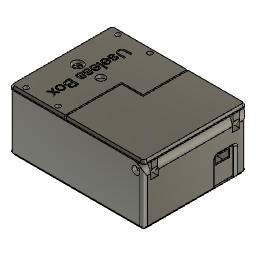
Smart_Useless_Box_box_v2 (Autodesk Fusion 360 design; units mm, degrees)
Autodesk Fusion 360 part; units mm, degrees
(part 1 of 2)
sketch "Base" plane through (0, 0, 0) normal (0, 0, 1) x (1, 0, 0) in component "Box Base"
  line L0 (50, -37.5) -> (-50, -37.5)
  line L1 (-50, -37.5) -> (-50, 37.5)
  line L2 (-50, 37.5) -> (50, 37.5)
  line L3 (50, 37.5) -> (50, -37.5)
  line L4 (50, -37.5) -> (-50, 37.5) construction
  line L5 (-50, -37.5) -> (50, 37.5) construction
  line L6 (50.5, -41) -> (-50.5, -41)
  line L7 (-53.5, -38) -> (-53.5, 38)
  line L8 (-50.5, 41) -> (50.5, 41)
  line L9 (53.5, 38) -> (53.5, -38)
  line L10 (53.5, -41) -> (-53.5, 41) construction
  line L11 (-53.5, -41) -> (53.5, 41) construction
  arc A0 (-53.5, -38) -> (-50.5, -41) centre (-50.5, -38) ccw
  arc A1 (-50.5, 41) -> (-53.5, 38) centre (-50.5, 38) ccw
  arc A2 (53.5, 38) -> (50.5, 41) centre (50.5, 38) ccw
  arc A3 (50.5, -41) -> (53.5, -38) centre (50.5, -38) ccw
  dimension "d5" = 100
  dimension "d6" = 75
  dimension "d7" = 82
  dimension "d8" = 107
  dimension "d9" = 3
  constraint perpendicular L0 L1
  constraint parallel L0 L2
  constraint parallel L1 L3
  constraint horizontal L0
  constraint coincident L4 origin
  constraint coincident L5 origin
  constraint perpendicular L6 L7
  constraint parallel L6 L8
  constraint parallel L7 L9
  constraint horizontal L6
  constraint coincident L10 origin
  constraint coincident L11 origin
  constraint coincident L11.start L6
  constraint coincident L11.start L7
  constraint tangent L6 A0
  constraint tangent L7 A0
  constraint coincident L10.end L7
  constraint coincident L10.end L8
  constraint tangent L7 A1
  constraint tangent L8 A1
  constraint equal A0 A1
  constraint coincident L11.end L8
  constraint coincident L11.end L9
  constraint tangent L8 A2
  constraint tangent L9 A2
  constraint equal A0 A2
  constraint coincident L10.start L9
  constraint coincident L10.start L6
  constraint tangent L9 A3
  constraint tangent L6 A3
  constraint equal A0 A3
  measures "d5" distance of L1.end L2.end
  measures "d6" distance of L0.end L1.end
  measures "d7" distance of L11.start L10.end
  measures "d8" distance of L10.end L11.end
  measures "d9" radius of A0
extrude "Extrude base bottom" add sketch "Base" along normal blind 2.4 contours L0 L1 L2 L3 makes body 1 in component "Box Base"
extrude "Extrude base wall" add sketch "Base" along normal blind 45 bodies 1 in component "Box Base"
chamfer "Chamfer bottom edges" distance 2 angle 35 8 edges at (-52.6213, -40.1213, 0) (-53.5, 0, 0) (-52.6213, 40.1213, 0) (0, 41, 0) (52.6213, 40.1213, 0) (53.5, 0, 0) (52.6213, -40.1213, 0) (0, -41, 0) measured on face at (-52.2402, -40.4437, 30) measured on face at (-16.8333, -13.6667, 0) measured on face at (-53.1665, 39.3747, 30) measured on face at (-16.8333, -13.6667, 0) measured on face at (52.9437, 39.7402, 30) measured on face at (-16.8333, -13.6667, 0) measured on face at (53.4966, -38.1427, 30) measured on face at (-16.8333, -13.6667, 0) on bodies 1 in component "Box Base"
ref_plane "WorkPlane1" through (-10, 0, 23.7) normal (1, 0, 0) x (0, 1, 0) in component "Box Base"
sketch "Lid mount profile" plane through (-10, 0, 23.7) normal (1, 0, 0) x (0, 1, 0) in component "Box Base"
  line L0 (-37.5, -21.3) -> (-37.5, 21.3)
  line L1 (-37.5, 21.3) -> (37.5, 21.3)
  line L2 (37.5, -21.3) -> (37.5, 21.3)
  line L3 (-32, 21.3) -> (-37.5, 13.4452)
  line L4 (32, 21.3) -> (37.5, 13.4452)
  dimension "d28" = 5.5
  dimension "d29" = 35
  dimension "d30" = 7.8548
  dimension "d31" = 5.5
  dimension "d32" = 35
  constraint coincident L1 L3.start
  constraint coincident L0 L3.end
  constraint coincident L1 L4.start
  constraint coincident L2 L4.end
  measures "d28" distance of L0.end L3.start
  measures "d29" angle of L0 L3
  measures "d30" distance of L0.end L3.end
  measures "d31" distance of L1.end L4.start
  measures "d32" angle of L2 L4
extrude "Extrude lid mount profiles" add sketch "Lid mount profile" against normal up to surface (40 mm away) bodies 1 in component "Box Base"
sketch "Lid mount screws" plane through (0, 0, 45) normal (0, 0, 1) x (-1, 0, 0) in component "Box Base"
  line L0 (10, -37.5) -> (-50, -37.5)
  line L1 (-50, -37.5) -> (-50, 37.5)
  line L2 (-50, 37.5) -> (10, 37.5)
  line L3 (10, 37.5) -> (10, 32)
  line L4 (10, 32) -> (50, 32)
  line L5 (50, 32) -> (50, -32)
  line L6 (50, -32) -> (10, -32)
  line L7 (10, -32) -> (10, -37.5)
  arc A0 (53.5, 38) -> (50.5, 41) centre (50.5, 38) ccw
  line L8 (50.5, 41) -> (-50.5, 41)
  arc A1 (-50.5, 41) -> (-53.5, 38) centre (-50.5, 38) ccw
  line L9 (-53.5, 38) -> (-53.5, -38)
  arc A2 (-53.5, -38) -> (-50.5, -41) centre (-50.5, -38) ccw
  line L10 (-50.5, -41) -> (50.5, -41)
  arc A3 (50.5, -41) -> (53.5, -38) centre (50.5, -38) ccw
  line L11 (53.5, -38) -> (53.5, 38)
  line L12 (44.5, -32) -> (44.5, -41) construction
  line L13 (44.5, -36.5) -> (19, -36.5) construction
  line L14 (53.5, 0) -> (-53.5, 0) construction
  circle A4 centre (44.5, -36.5) radius 1.5
  circle A5 centre (19, -36.5) radius 1.5
  circle A6 centre (19, 36.5) radius 1.5
  circle A7 centre (44.5, 36.5) radius 1.5
  dimension "d36" = 9
  dimension "d37" = 9
  dimension "d38" = 3
  dimension "d39" = 3
  constraint coincident L6 L12.start
  constraint coincident L10 L12.end
  constraint perpendicular L10 L12
  constraint midpoint L12 L13.start
  constraint perpendicular L12 L13
  constraint midpoint L11 L14.start
  constraint midpoint L9 L14.end
  constraint coincident L13.start A4.centre
  constraint coincident L13.end A5.centre
  constraint symmetric L14 A4 A7
  constraint symmetric L14 A5 A6
  measures "d36" distance of L11 L12
  measures "d37" distance of L7 L13.end
  measures "d38" diameter of A4
  measures "d39" diameter of A5
extrude "Extrude5" cut sketch "Lid mount screws" against normal blind 15 contours A4 | A5 | A6 | A7 bodies 1 in component "Box Base"
chamfer "Chamfer screw hole edges" distance 1 angle 45 4 edges at (-43.1015, 35.9576, 45) (-17.6015, 35.9576, 45) (-43.1015, -37.0424, 45) (-17.6015, -37.0424, 45) on bodies 1 in component "Box Base"
sketch "Board support" plane through (0, 0, 2.4) normal (0, 0, 1) x (-1, 0, 0) in component "Box Base"
  line L0 (-50, -37.5) -> (50, -37.5)
  line L1 (50, -37.5) -> (50, 37.5)
  line L2 (50, 37.5) -> (-50, 37.5)
  line L3 (-50, 37.5) -> (-50, -37.5)
  line L4 (-50, -37.5) -> (-49.99, -37.5)
  line L5 (-49.99, -37.5) -> (-49.99, -11)
  line L6 (-49.99, -11) -> (-50, -11)
  line L7 (-50, -11) -> (-50, -37.5)
  line L8 (-49.99, -37.5) -> (-49.98, -37.5)
  line L9 (-49.98, -10.99) -> (-50, -10.99)
  line L10 (-50, -11) -> (-50, -10.99)
  line L11 (-49.98, -10.99) -> (-49.98, -37.5)
  line L12 (-50, -37.5) -> (-50, -11)
  dimension "d50" = 0.01
  dimension "d51" = 26.5
  dimension "d52" = 0.01
  dimension "d53" = 0.01
  dimension "d56" = 0.01
  constraint horizontal L4
  constraint vertical L5
  constraint horizontal L6
  constraint vertical L7
  constraint coincident L0.start L3.end
  constraint coincident L0 L8.end
  constraint perpendicular L5 L8
  constraint coincident L3 L9.end
  constraint perpendicular L3 L9
  constraint perpendicular L8 L11
  constraint coincident L4 L0.start
  constraint coincident L6 L7.start
  constraint perpendicular L6 L12
  measures "d50" distance of L0.start L4.end
  measures "d51" distance of L0.start L6.end
  measures "d52" distance of L4.end L8.end
  measures "d53" distance of L6 L9
  measures "d56" distance of L5 L12
extrude "Extrude board base support" add sketch "Board support" along normal blind 0.01 contours L0 L3 L4 L5 L6 L7 L12 bodies 1 in component "Box Base"
extrude "Extrude board wall support" add sketch "Board support" along normal blind 0.01 contours L0 L3 L5 L6 L8 L9 L10 L11 bodies 1 in component "Box Base"
sketch "USB hole" plane through (53.5, 0, 0) normal (1, 0, 0) x (0, 1, 0) in component "Box Base"
  line L0 (-38, 2) -> (38, 2)
  line L1 (38, 2) -> (38, 45)
  line L2 (38, 45) -> (-38, 45)
  line L3 (-38, 45) -> (-38, 2)
  line L4 (11, 2.4) -> (37.5, 2.4)
  line L5 (29.75, 2.4) -> (18.75, 2.4)
  line L6 (18.75, 2.4) -> (18.75, 20.4)
  line L7 (18.75, 20.4) -> (29.75, 20.4)
  line L8 (29.75, 20.4) -> (29.75, 2.4)
  line L9 (29.75, 2.4) -> (18.75, 20.4) construction
  line L10 (18.75, 2.4) -> (29.75, 20.4) construction
  line L11 (31.75, 0.4) -> (16.75, 0.4)
  line L12 (16.75, 0.4) -> (16.75, 21.4)
  line L13 (17.75, 22.4) -> (30.75, 22.4)
  line L14 (31.75, 21.4) -> (31.75, 0.4)
  line L15 (31.75, 0.4) -> (16.75, 22.4) construction
  line L16 (16.75, 0.4) -> (31.75, 22.4) construction
  arc A0 (17.75, 22.4) -> (16.75, 21.4) centre (17.75, 21.4) ccw
  arc A1 (31.75, 21.4) -> (30.75, 22.4) centre (30.75, 21.4) ccw
  point P0 (24.25, 11.4)
  point P1 (24.25, 11.4)
  dimension "d69" = 11
  dimension "d70" = 18
  dimension "d71" = 15
  dimension "d72" = 22
  dimension "d73" = 1
  constraint perpendicular L5 L6
  constraint parallel L5 L7
  constraint parallel L6 L8
  constraint horizontal L5
  constraint coincident L9 P1
  constraint coincident L10 P1
  constraint midpoint L4 L5
  constraint perpendicular L11 L12
  constraint parallel L11 L13
  constraint parallel L12 L14
  constraint horizontal L11
  constraint coincident L15 P1
  constraint coincident L16 P1
  constraint coincident P1 P0
  constraint coincident L15.end L12
  constraint coincident L15.end L13
  constraint tangent L12 A0
  constraint tangent L13 A0
  constraint coincident L16.end L13
  constraint coincident L16.end L14
  constraint tangent L13 A1
  constraint tangent L14 A1
  constraint equal A0 A1
  measures "d69" distance of L6.end L7.end
  measures "d70" distance of L5.end L6.end
  measures "d71" distance of L15.end L16.end
  measures "d72" distance of L11.end L15.end
  measures "d73" radius of A0
extrude "Cut USB hole" cut sketch "USB hole" against normal up to surface (3.5 mm away) contours L4 L5 L6 L7 L8 bodies 1 in component "Box Base"
extrude "Cut USB cable hole" cut sketch "USB hole" against normal blind 2.5 contours L0 L4 L5 L12 L14 | L0 L11 L12 L14 | L4 L6 L7 L8 L12 L13 L14 A0 A1 bodies 1 in component "Box Base"
chamfer "Chamfer USB edges" distance 2 angle 35 5 edges at (53.5, 16.75, 11.7) (53.5, 17.0429, 22.1071) (53.5, 24.25, 22.4) (53.5, 31.4571, 22.1071) (53.5, 31.75, 11.7) measured on face at (53.5, -19.75, 22.8) measured on face at (53.5, -19.75, 22.8) measured on face at (53.5, -19.75, 22.8) measured on face at (53.5, -19.75, 22.8) measured on face at (53.5, -19.75, 22.8) on bodies 1 in component "Box Base"
sketch "Shaft" plane through (0, -41, 0) normal (0, -1, 0) x (1, 0, 0) in component "Box Base"
  line L0 (-50.5, 2) -> (50.5, 2)
  line L1 (50.5, 2) -> (50.5, 45)
  line L2 (50.5, 45) -> (-50.5, 45)
  line L3 (-50.5, 45) -> (-50.5, 2)
  line L4 (53.5, 21.4) -> (53.5, 2)
  line L5 (53.5, 2) -> (53.5, 45)
  line L6 (53.5, 45) -> (53.5, 2)
  line L7 (53.5, 2) -> (53.5, 21.4)
  line L8 (53.5, 21.4) -> (53.5, 24.4)
  line L9 (53.5, 21.4) -> (53.5, 24.4)
  line L10 (-10, 45) -> (50, 45)
  line L11 (50, 2.41) -> (50, 45)
  circle A0 centre (47.3, 38.8) radius 1.5
  circle A1 centre (47.3, 38.8) radius 3.2
  circle A2 centre (47.3, 38.8) radius 6.2
  line L12 (41.1, 38.8) -> (41.1, 45)
  line L13 (42.2213, 35.2438) -> (50, 24.1346)
  spline S0 degree 5 poles (45.3, 45) (45.5877, 44.9597) (46.1522, 44.8682) (46.9666, 44.6986) (47.9866, 44.4066) (49.1443, 43.9243) (50.1744, 43.3144) (51.0663, 42.5663) (51.8144, 41.6744) (52.4243, 40.6443) (52.9066, 39.4866) (53.1986, 38.4666) (53.3682, 37.6522) (53.4597, 37.0877) (53.5, 36.8) knots 0 0 0 0 0 0 0.1 0.2 0.3 0.4 0.5 0.6 0.7 0.8 0.9 1 1 1 1 1 1
  line L14 (47.3, 38.8) -> (53.5, 45) construction
  line L15 (53.5, 45) -> (50, 45)
  point P0 (51.0304, 42.5304)
  dimension "d99" = 3
  dimension "d100" = 6.4
  dimension "d101" = 12.4
  dimension "d103" = 6.2
  dimension "d104" = 6.2
  dimension "d105" = 35
  dimension "d123" = 8.2
  dimension "d124" = 8.2
  constraint concentric A0 A1
  constraint concentric A0 A2
  constraint coincident A2 L12.start
  constraint tangent A2 L12
  constraint coincident L10 L12.end
  constraint perpendicular L2 L12
  constraint coincident A2 L13.start
  constraint tangent A2 L13
  constraint coincident L11 L13.end
  constraint coincident L10 S0.start
  constraint coincident L5 S0.end
  constraint coincident A0.centre A1.centre
  constraint coincident L5.end L6.start
  constraint coincident P0 L14
  constraint coincident L10.end L11.end
  measures "d99" diameter of A0
  measures "d100" diameter of A1
  measures "d101" diameter of A2
  measures "d103" distance of L2 A0.centre
  measures "d104" distance of L6 A0.centre
  measures "d105" angle of L11 L13
  measures "d123" distance of S0.start L5.end
  measures "d124" distance of S0.end L5.end
extrude "Extrude20" cut sketch "Shaft" against normal up to surface (82 mm away) contours L1 A2 S0 | L5 L6 A2 S0 | L1 L11 A2 S0 | L1 L5 L6 A2 L15 | L2 L10 A2 S0 | L1 L2 L11 A2 L15 | L11 A2 S0 | L2 L10 L11 A2 picked at (52.3629, 41.2358) bodies 1 in component "Box Base"
extrude "Extrude shaft case" add sketch "Shaft" against normal up to surface (78.5 mm away) contours L11 A1 A2 S0 | L11 A2 L13 | L2 L10 A2 L12 S0 | L11 A1 | L2 L10 A2 S0 | L11 A2 S0 | L2 L10 L11 A2 | A0 picked at (49.6, 38.8) bodies 1 in component "Box Base"
extrude "Cut shaft screw hole" cut sketch "Shaft" against normal up to surface (82 mm away) contours A0 bodies 1 in component "Box Base"
extrude "Cut shaft screw head hole front" cut sketch "Shaft" against normal blind 3.5 contours L11 A1 | L11 A1 bodies 1 in component "Box Base"
sketch "Shaft head hole back" plane through (0, 41, 0) normal (0, 1, 0) x (-1, 0, 0) in component "Box Base"
  circle A0 centre (-47.3, 38.8) radius 1.5
  line L0 (-50.5, 2) -> (50.5, 2)
  line L1 (50.5, 2) -> (50.5, 45)
  line L2 (50.5, 45) -> (-45.3, 45)
  line L3 (-50.5, 43.0074) -> (-50.5, 2)
  circle A1 centre (-47.3, 38.8) radius 3.2
  spline S0 degree 5 poles (-45.3, 45) (-45.5877, 44.9597) (-46.1522, 44.8682) (-46.9666, 44.6986) (-47.9866, 44.4066) (-49.0021, 43.9836) (-49.7129, 43.5838) (-50.175, 43.2634) (-50.43, 43.0639) (-50.5, 43.0074) knots 0 0 0 0 0 0 0.1 0.2 0.3 0.4 0.438574 0.438574 0.438574 0.438574 0.438574 0.438574
extrude "Cut shaft screw head hole back" cut sketch "Shaft head hole back" against normal blind 3.5 contours A1 bodies 1 in component "Box Base"
sketch "Shaft top mount holes" plane through (0, 0, 45) normal (0, 0, 1) x (-1, 0, 0) in component "Box Base"
  line L0 (50.5, 41) -> (-50, 41)
  line L1 (-45.3, -41) -> (50.5, -41)
  arc A0 (50.5, -41) -> (53.5, -38) centre (50.5, -38) ccw
  line L2 (53.5, -38) -> (53.5, 38)
  arc A1 (53.5, 38) -> (50.5, 41) centre (50.5, 38) ccw
  line L3 (-41.1, 37.5) -> (10, 37.5)
  line L4 (10, 37.5) -> (10, 32)
  line L5 (10, 32) -> (50, 32)
  line L6 (50, 32) -> (50, -32)
  line L7 (50, -32) -> (10, -32)
  line L8 (10, -32) -> (10, -37.5)
  line L9 (10, -37.5) -> (-41.1, -37.5)
  line L10 (-41.1, -37.5) -> (-41.1, 37.5)
  circle A2 centre (44.5, 36.5) radius 2.5
  circle A3 centre (44.5, -36.5) radius 2.5
  circle A4 centre (19, -36.5) radius 2.5
  circle A5 centre (19, 36.5) radius 2.5
  line L11 (-41.1, -35.5) -> (-53.5, -35.5)
  line L12 (-53.5, -35.5) -> (-53.5, -29.5)
  line L13 (-53.5, -29.5) -> (-41.1, -29.5)
  line L14 (-41.1, -29.5) -> (-41.1, -35.5)
  line L15 (-45.3, -37.5) -> (-45.3, -41)
  line L16 (-50, 41) -> (-50, -37.5)
  line L17 (-50, -37.5) -> (-45.3, -37.5)
  line L18 (53.5, 0) -> (-50, 0) construction
  line L19 (-41.1, 35.5) -> (-53.5, 35.5)
  line L20 (-53.5, 35.5) -> (-53.5, 29.5)
  line L21 (-53.5, 29.5) -> (-41.1, 29.5)
  line L22 (-41.1, 29.5) -> (-41.1, 35.5)
  dimension "d115" = 6
  dimension "d130" = 2
  constraint horizontal L11
  constraint vertical L12
  constraint horizontal L13
  constraint vertical L14
  constraint midpoint L2 L18.start
  constraint coincident L16 L18.end
  constraint perpendicular L16 L18
  constraint symmetric L11.start L18 L19.start
  constraint symmetric L11.end L18 L19.end
  constraint symmetric L12.end L18 L20.end
  constraint symmetric L13.end L18 L21.end
  measures "d115" distance of L11 L13
  measures "d130" distance of L11 L15.start
extrude "Cut shaft top mount holes" cut sketch "Shaft top mount holes" against normal blind 12.4 contours L10 L16 L19 L21 L22 | L16 L19 L20 L21 | L11 L12 L13 L16 | L10 L11 L13 L14 L16 bodies 1 in component "Box Base"
extrude "Cut shaft roundover" cut sketch "Shaft" against normal up to surface (82 mm away) contours L1 A2 S0 | L5 L6 A2 S0 | L1 L11 A2 S0 | L1 L5 L6 A2 L15 | L2 L10 A2 S0 | L1 L2 L11 A2 L15 | L11 A2 S0 | L2 L10 L11 A2 picked at (52.3629, 41.2358) bodies 1 in component "Box Base"
sketch "Top" plane through (0, 0, 45) normal (0, 0, 1) x (-1, 0, 0) in component "Fixed Lid"
  circle A0 centre (44.5, 36.5) radius 2.5
  circle A1 centre (44.5, -36.5) radius 2.5
  circle A2 centre (19, -36.5) radius 2.5
  circle A3 centre (19, 36.5) radius 2.5
  line L0 (-45.3, 41) -> (-45.3, 35.5)
  line L1 (-45.3, 35.5) -> (-41.1, 35.5)
  line L2 (-41.1, 35.5) -> (-41.1, 37.5)
  line L3 (-41.1, 37.5) -> (10, 37.5)
  line L4 (10, 37.5) -> (10, 32)
  line L5 (10, 32) -> (50, 32)
  line L6 (50, 32) -> (50, -32)
  line L7 (50, -32) -> (10, -32)
  line L8 (10, -32) -> (10, -37.5)
  line L9 (10, -37.5) -> (-41.1, -37.5)
  line L10 (-41.1, -37.5) -> (-41.1, -35.5)
  line L11 (-41.1, -35.5) -> (-45.3, -35.5)
  line L12 (-45.3, -35.5) -> (-45.3, -41)
  line L13 (-45.3, -41) -> (50.5, -41)
  arc A4 (50.5, -41) -> (53.5, -38) centre (50.5, -38) ccw
  line L14 (53.5, -38) -> (53.5, 38)
  arc A5 (53.5, 38) -> (50.5, 41) centre (50.5, 38) ccw
  line L15 (50.5, 41) -> (-45.3, 41)
  line L16 (10, -41) -> (10, 41)
  circle A6 centre (19, -36.5) radius 1.9
  circle A7 centre (44.5, -36.5) radius 1.9
  circle A8 centre (44.5, 36.5) radius 1.9
  circle A9 centre (19, 36.5) radius 1.9
  line L17 (0, 0) -> (53.5, 0) construction
  circle A10 centre (21.5, 0) radius 3.35
  line L18 (-7, -41) -> (-7, -5)
  line L19 (-7, -5) -> (10, -5)
  circle A11 centre (40, 0) radius 3.1
  line L20 (48, -5) -> (32, -5)
  line L21 (32, -5) -> (32, 16)
  line L22 (32, 16) -> (48, 16)
  line L23 (48, 16) -> (48, -5)
  line L24 (50, 18) -> (50, -7)
  line L25 (50, -7) -> (30, -7)
  line L26 (30, -7) -> (30, 18)
  line L27 (30, 18) -> (50, 18)
  line L28 (50, -32) -> (50, 32) construction
  line L29 (40, -5) -> (40, 16) construction
  dimension "d132" = 3.8
  dimension "d133" = 3.8
  dimension "d134" = 3.8
  dimension "d135" = 3.8
  dimension "d138" = 6.7
  dimension "d140" = 11.5
  dimension "d143" = 17
  dimension "d145" = 5
  dimension "d152" = 6.2
  dimension "d156" = 16
  dimension "d157" = 21
  dimension "d160" = 5
  constraint coincident L13 L16.start
  constraint coincident L15 L16.end
  constraint perpendicular L15 L16
  constraint collinear L8 L16
  constraint concentric A2 A6
  constraint concentric A1 A7
  constraint concentric A0 A8
  constraint concentric A3 A9
  constraint coincident L17.start origin
  constraint midpoint L14 L17.end
  constraint coincident L17 A10.centre
  constraint coincident L13 L18.start
  constraint perpendicular L13 L18
  constraint coincident L16 L19.end
  constraint perpendicular L16 L19
  constraint coincident L17 A11.centre
  constraint horizontal L20
  constraint vertical L21
  constraint horizontal L22
  constraint vertical L23
  constraint coincident L6.end L7.start
  constraint coincident L5.end L6.start
  constraint coincident L24 L5.end
  constraint midpoint L20 L29.start
  constraint midpoint L22 L29.end
  constraint coincident A11.centre L29
  measures "d132" diameter of A6
  measures "d133" diameter of A7
  measures "d134" diameter of A8
  measures "d135" diameter of A9
  measures "d138" diameter of A10
  measures "d140" distance of L16 A10.centre
  measures "d143" distance of L16 L18
  measures "d145" distance of L17.start L19
  measures "d152" diameter of A11
  measures "d156" distance of L20.start L20.end
  measures "d157" distance of L20.start L22.end
  measures "d160" distance of A11.centre L20
extrude "Extrude fixed lid" add sketch "Top" along normal blind 2.6 separate body contours A0 | A1 | A2 | A3 | L4 L5 L6 L7 L8 L13 A4 L14 A5 L15 L16 L24 | L5 L6 L7 L16 L25 L26 L27 | L8 L9 L16 L18 L19 | L6 L24 L25 L26 L27 | L9 L13 L16 L18 | L20 L21 L22 L23 makes body 2 in component "Fixed Lid"
chamfer "Chamfer1" distance 1.2 angle 55 6 edges at (-21.75, 41, 47.6) (-52.6213, 40.1213, 47.6) (-53.5, 0, 47.6) (-52.6213, -40.1213, 47.6) (-30.25, -41, 47.6) (-37.1098, -1.121, 47.6) measured on face at (-6.8691, 25.9026, 47.6) measured on face at (-6.8691, 25.9026, 47.6) measured on face at (-6.8691, 25.9026, 47.6) measured on face at (-6.8691, 25.9026, 47.6) measured on face at (-6.8691, 25.9026, 47.6) measured on face at (-6.8691, 25.9026, 47.6) on bodies 2 in component "Fixed Lid"
sketch "Bottom" plane through (0, 0, 45) normal (0, 0, -1) x (1, 0, 0) in component "Fixed Lid"
  circle A0 centre (-21.5, 0) radius 3.35
  circle A1 centre (-40, 0) radius 3.1
  circle A2 centre (-19, 36.5) radius 1.9
  circle A3 centre (-44.5, 36.5) radius 1.9
  circle A4 centre (-44.5, -36.5) radius 1.9
  circle A5 centre (-19, -36.5) radius 1.9
  line L0 (-50.5, -41) -> (7, -41)
  line L1 (7, -41) -> (7, -5)
  line L2 (7, -5) -> (-10, -5)
  line L3 (-10, -5) -> (-10, 41)
  line L4 (-10, 41) -> (-50.5, 41)
  arc A6 (-50.5, 41) -> (-53.5, 38) centre (-50.5, 38) ccw
  line L5 (-53.5, 38) -> (-53.5, -38)
  arc A7 (-53.5, -38) -> (-50.5, -41) centre (-50.5, -38) ccw
  line L6 (-50, -7) -> (-30, -7)
  line L7 (-30, -7) -> (-30, 18)
  line L8 (-50, 18) -> (-50, -7)
  line L9 (-30, 18) -> (-50, 18)
  line L10 (-48, -5) -> (-32, -5)
  line L11 (-32, -5) -> (-32, 16)
  line L12 (-48, 16) -> (-48, -5)
  line L13 (-32, 16) -> (-48, 16)
  line L14 (7, -41) -> (7, -5)
  line L15 (7, -23.5) -> (1.6, -23.5)
  line L16 (1.6, -23.5) -> (1.6, -15)
  line L17 (1.6, -15) -> (7, -15)
  line L18 (7, -15) -> (7, -23.5)
  line L19 (-21.6, -23.5) -> (-27, -23.5)
  line L20 (-27, -23.5) -> (-27, -15)
  line L21 (-27, -15) -> (-21.6, -15)
  line L22 (-21.6, -15) -> (-21.6, -23.5)
  line L23 (-42.6, -5) -> (-48, -5)
  line L24 (-48, -5) -> (-48, 0.4)
  line L25 (-48, 0.4) -> (-42.6, 0.4)
  line L26 (-42.6, 0.4) -> (-42.6, -5)
  line L27 (-42.6, -5) -> (-48, 0.4) construction
  line L28 (-48, -5) -> (-42.6, 0.4) construction
  line L29 (-32, -5) -> (-37.4, -5)
  line L30 (-37.4, -5) -> (-37.4, 0.4)
  line L31 (-37.4, 0.4) -> (-32, 0.4)
  line L32 (-32, 0.4) -> (-32, -5)
  line L33 (-32, -5) -> (-37.4, 0.4) construction
  line L34 (-37.4, -5) -> (-32, 0.4) construction
  circle A8 centre (-45.3, -2.3) radius 1.25
  circle A9 centre (-34.7, -2.3) radius 1.25
  arc A10 (-42.6, -2.3) -> (-45.3, 0.4) centre (-45.3, -2.3) ccw
  arc A11 (-34.7, 0.4) -> (-37.4, -2.3) centre (-34.7, -2.3) ccw
  point P0 (-45.3, -2.3)
  point P1 (-34.7, -2.3)
  dimension "d170" = 15
  dimension "d171" = 8.5
  dimension "d172" = 5.4
  dimension "d173" = 15
  dimension "d174" = 8.5
  dimension "d175" = 5.4
  dimension "d176" = 23.2
  dimension "d192" = 5.4
  dimension "d193" = 5.4
  dimension "d194" = 5.4
  dimension "d195" = 5.4
  dimension "d196" = 2.5
  dimension "d197" = 2.5
  constraint horizontal L15
  constraint vertical L16
  constraint horizontal L17
  constraint vertical L18
  constraint coincident L14 L15.start
  constraint horizontal L19
  constraint vertical L20
  constraint horizontal L21
  constraint vertical L22
  constraint perpendicular L23 L24
  constraint parallel L23 L25
  constraint parallel L24 L26
  constraint horizontal L23
  constraint coincident L27 P0
  constraint coincident L28 P0
  constraint coincident L10.start L12.end
  constraint perpendicular L29 L30
  constraint parallel L29 L31
  constraint parallel L30 L32
  constraint horizontal L29
  constraint coincident L33 P1
  constraint coincident L34 P1
  constraint coincident L10.end L11.start
  constraint coincident P0 A8.centre
  constraint coincident P1 A9.centre
  constraint midpoint L26 A10.start
  constraint midpoint L25 A10.end
  constraint midpoint L30 A11.end
  constraint midpoint L31 A11.start
  measures "d170" distance of origin L17
  measures "d171" distance of L15.end L16.end
  measures "d172" distance of L15.start L15.end
  measures "d173" distance of origin L21
  measures "d174" distance of L19.end L20.end
  measures "d175" distance of L19.start L19.end
  measures "d176" distance of L16 L22
  measures "d192" distance of L24.end L25.end
  measures "d193" distance of L10.start L24.end
  measures "d194" distance of L30.end L31.end
  measures "d195" distance of L29.end L30.end
  measures "d196" diameter of A8
  measures "d197" diameter of A9
extrude "Extrude6" add sketch "Bottom" along normal blind 1.6 contours A1 L10 L11 L29 L30 L31 L32 A11 | A1 A11 | A1 A10 | A1 L10 L12 L23 L24 L25 L26 A10 bodies 2 in component "Fixed Lid"
extrude "Extrude motor mounts" add sketch "Bottom" along normal blind 13 contours L1 L14 L15 L16 L17 L18 | L19 L20 L21 L22 bodies 2 in component "Fixed Lid"
extrude "Extrude sensor wall support" add sketch "Bottom" along normal blind 4 contours L6 L7 L8 L9 bodies 2 in component "Fixed Lid"
sketch "Motor mounts" plane through (0, 15, 0) normal (0, -1, 0) x (1, 0, 0) in component "Fixed Lid"
  line L0 (7, 45) -> (1.6, 45)
  line L1 (1.6, 45) -> (1.6, 32)
  line L2 (1.6, 32) -> (7, 32)
  line L3 (7, 32) -> (7, 45)
  line L4 (-21.6, 45) -> (-27, 45)
  line L5 (-27, 45) -> (-27, 32)
  line L6 (-27, 32) -> (-21.6, 32)
  line L7 (-21.6, 32) -> (-21.6, 45)
  line L8 (-24.3, 45) -> (-24.3, 32) construction
  line L9 (4.3, 45) -> (4.3, 32) construction
  circle A0 centre (-24.3, 38.7) radius 1.1
  circle A1 centre (4.3, 38.7) radius 1.1
  line L10 (-27, 45) -> (-21.6, 45)
  line L11 (1.6, 45) -> (7, 45)
  dimension "d179" = 2.2
  dimension "d180" = 2.2
  dimension "d182" = 6.3
  dimension "d183" = 6.3
  constraint midpoint L4 L8.start
  constraint midpoint L6 L8.end
  constraint midpoint L0 L9.start
  constraint midpoint L2 L9.end
  constraint coincident L8 A0.centre
  constraint coincident L9 A1.centre
  measures "d179" diameter of A0
  measures "d180" diameter of A1
  measures "d182" distance of A0.centre L10
  measures "d183" distance of A1.centre L11
extrude "Cut motor mount holes" cut sketch "Motor mounts" against normal up to surface (8.5 mm away) contours A0 | A1 bodies 2 in component "Fixed Lid"
fillet "Fillet1" radius 4 3 edges at (-27, 19.25, 45) (-24.3, 23.5, 45) (4.3, 23.5, 45) on bodies 2 in component "Fixed Lid"
sketch "Text" plane through (0, 0, 47.6) normal (0, 0, 1) x (-1, 0, 0) in component "Fixed Lid"
  circle A0 centre (21.5, 0) radius 3.35
  circle A1 centre (19, 36.5) radius 1.9
  circle A2 centre (44.5, 36.5) radius 1.9
  circle A3 centre (44.5, -36.5) radius 1.9
  circle A4 centre (19, -36.5) radius 1.9
  line L0 (-7, -39.8) -> (50.5, -39.8)
  arc A5 (50.5, -39.8) -> (52.3, -38) centre (50.5, -38) ccw
  line L1 (52.3, -38) -> (52.3, 38)
  arc A6 (52.3, 38) -> (50.5, 39.8) centre (50.5, 38) ccw
  line L2 (50.5, 39.8) -> (10, 39.8)
  line L3 (10, 39.8) -> (10, -5)
  line L4 (10, -5) -> (-7, -5)
  line L5 (-7, -5) -> (-7, -39.8)
  circle A7 centre (40, 0) radius 4.3
  line L6 (33.8228, -28.9087) -> (33.8228, 31.2798) construction
  line L7 (33.8228, 31.2798) -> (22.8228, 31.2798) construction
  line L8 (22.8228, 31.2798) -> (22.8228, -28.9087) construction
  line L9 (22.8228, -28.9087) -> (33.8228, -28.9087) construction
  text T0 "Useless Box" font "Arial" height 11 align ink ink in box 0 x 0 at (33.8228, -28.9087) x (0, 1) y (-1, 0) spacing 1 height is em
  constraint perpendicular L6 L7
  constraint parallel L6 L8
  constraint parallel L7 L9
extrude "Extrude5'" cut sketch "Text" against normal blind 1 text T0 bodies 2 in component "Fixed Lid"
sketch "Bottom (2)" plane through (0, 0, 45) normal (0, 0, 1) x (-1, 0, 0) in component "Moving Lid"
  circle A0 centre (44.5, 36.5) radius 2.5
  circle A1 centre (44.5, -36.5) radius 2.5
  circle A2 centre (19, -36.5) radius 2.5
  circle A3 centre (19, 36.5) radius 2.5
  line L0 (-45.3, 41) -> (-45.3, 35.5)
  line L1 (-45.3, 35.5) -> (-41.1, 35.5)
  line L2 (-41.1, 35.5) -> (-41.1, 37.5)
  line L3 (-41.1, 37.5) -> (10, 37.5)
  line L4 (10, 37.5) -> (10, 32)
  line L5 (10, 32) -> (50, 32)
  line L6 (50, 32) -> (50, -32)
  line L7 (50, -32) -> (10, -32)
  line L8 (10, -32) -> (10, -37.5)
  line L9 (10, -37.5) -> (-41.1, -37.5)
  line L10 (-41.1, -37.5) -> (-41.1, -35.5)
  line L11 (-41.1, -35.5) -> (-45.3, -35.5)
  line L12 (-45.3, -35.5) -> (-45.3, -41)
  line L13 (-45.3, -41) -> (50.5, -41)
  arc A4 (50.5, -41) -> (53.5, -38) centre (50.5, -38) ccw
  line L14 (53.5, -38) -> (53.5, 38)
  arc A5 (53.5, 38) -> (50.5, 41) centre (50.5, 38) ccw
  line L15 (50.5, 41) -> (-45.3, 41)
  circle A6 centre (40, 0) radius 4.3
  line L16 (-7, -39.8) -> (50.5, -39.8)
  arc A7 (50.5, -39.8) -> (52.3, -38) centre (50.5, -38) ccw
  line L17 (52.3, -38) -> (52.3, 38)
  arc A8 (52.3, 38) -> (50.5, 39.8) centre (50.5, 38) ccw
  line L18 (50.5, 39.8) -> (10, 39.8)
  line L19 (10, 39.8) -> (10, -5)
  line L20 (10, -5) -> (-7, -5)
  line L21 (-7, -5) -> (-7, -39.8)
  circle A9 centre (19, 36.5) radius 1.9
  circle A10 centre (44.5, -36.5) radius 1.9
  circle A11 centre (19, -36.5) radius 1.9
  circle A12 centre (21.5, 0) radius 3.35
  circle A13 centre (44.5, 36.5) radius 1.9
  spline S0 degree 3 poles (32.3472, -24.2366) (32.0988, -24.0953) (31.4834, -23.7453) (30.7695, -23.7469) (30.3438, -23.7478) knots 0 0 0 0 0.084501 0.209307 0.209307 0.209307 0.209307
  line L22 (30.3438, -23.7478) -> (25.7998, -23.7478)
  line L23 (25.7998, -23.7478) -> (25.7998, -22.7058)
  line L24 (25.7998, -22.7058) -> (30.3492, -22.7058)
  spline S1 degree 3 poles (30.3492, -22.7058) (30.7068, -22.7108) (31.3475, -22.7197) (31.9626, -22.8963) (32.2344, -22.9744) knots 0 0 0 0 0.106693 0.191173 0.191173 0.191173 0.191173
  spline S2 degree 3 poles (32.2344, -22.9744) (32.4583, -23.0852) (32.9192, -23.3131) (33.219, -23.7315) (33.3731, -23.9465) knots 0 0 0 0 0.07376 0.151783 0.151783 0.151783 0.151783
  spline S3 degree 3 poles (33.3731, -23.9465) (33.4997, -24.2115) (33.7767, -24.7909) (33.7971, -25.4343) (33.8081, -25.7835) knots 0 0 0 0 0.087172 0.190602 0.190602 0.190602 0.190602
  spline S4 degree 3 poles (33.8081, -25.7835) (33.7983, -26.1236) (33.7802, -26.7511) (33.5378, -27.3289) (33.4268, -27.5935) knots 0 0 0 0 0.101025 0.186391 0.186391 0.186391 0.186391
  spline S5 degree 3 poles (33.4268, -27.5935) (33.2864, -27.8109) (33.0076, -28.2427) (32.552, -28.4801) (32.3257, -28.5979) knots 0 0 0 0 0.076197 0.151336 0.151336 0.151336 0.151336
  spline S6 degree 3 poles (32.3257, -28.5979) (32.0422, -28.6853) (31.3993, -28.8835) (30.7257, -28.8932) (30.3492, -28.8987) knots 0 0 0 0 0.088589 0.200829 0.200829 0.200829 0.200829
  line L25 (30.3492, -28.8987) -> (25.7998, -28.8987)
  line L26 (25.7998, -28.8987) -> (25.7998, -27.8567)
  line L27 (25.7998, -27.8567) -> (30.3438, -27.8567)
  spline S7 degree 3 poles (30.3438, -27.8567) (30.643, -27.8556) (31.1563, -27.8538) (31.6518, -27.7232) (31.8584, -27.6687) knots 0 0 0 0 0.089284 0.153164 0.153164 0.153164 0.153164
  spline S8 degree 3 poles (31.8584, -27.6687) (32.0106, -27.5926) (32.3168, -27.4396) (32.5086, -27.156) (32.605, -27.0134) knots 0 0 0 0 0.050134 0.100841 0.100841 0.100841 0.100841
  spline S9 degree 3 poles (32.605, -27.0134) (32.6817, -26.8433) (32.8447, -26.4817) (32.8601, -26.0849) (32.8682, -25.8748) knots 0 0 0 0 0.055462 0.117846 0.117846 0.117846 0.117846
  spline S10 degree 3 poles (32.8682, -25.8748) (32.8605, -25.5342) (32.847, -24.9324) (32.4985, -24.4472) (32.3472, -24.2366) knots 0 0 0 0 0.099283 0.175461 0.175461 0.175461 0.175461
  spline S11 degree 3 poles (33.0079, -13.1936) (32.9979, -13.0252) (32.9786, -12.6994) (32.81, -12.4206) (32.7286, -12.2859) knots 0 0 0 0 0.049772 0.096252 0.096252 0.096252 0.096252
  spline S12 degree 3 poles (32.7286, -12.2859) (32.6139, -12.1645) (32.3629, -11.8985) (32.0221, -11.7632) (31.837, -11.6897) knots 0 0 0 0 0.049501 0.108413 0.108413 0.108413 0.108413
  line L28 (31.837, -11.6897) -> (31.9605, -10.6907)
  spline S13 degree 3 poles (31.9605, -10.6907) (32.2331, -10.7825) (32.7605, -10.9601) (33.1373, -11.3687) (33.3194, -11.5662) knots 0 0 0 0 0.084738 0.163983 0.163983 0.163983 0.163983
  spline S14 degree 3 poles (33.3194, -11.5662) (33.4602, -11.8026) (33.7593, -12.3046) (33.7877, -12.8896) (33.8028, -13.199) knots 0 0 0 0 0.081309 0.172615 0.172615 0.172615 0.172615
  spline S15 degree 3 poles (33.8028, -13.199) (33.7771, -13.5884) (33.7279, -14.3331) (33.2586, -14.9107) (33.0347, -15.1863) knots 0 0 0 0 0.113886 0.217791 0.217791 0.217791 0.217791
  spline S16 degree 3 poles (33.0347, -15.1863) (32.7361, -15.399) (32.091, -15.8586) (31.2967, -15.8964) (30.8702, -15.9168) knots 0 0 0 0 0.107752 0.232763 0.232763 0.232763 0.232763
  spline S17 degree 3 poles (30.8702, -15.9168) (30.4295, -15.8967) (29.6116, -15.8593) (28.9438, -15.3914) (28.6358, -15.1755) knots 0 0 0 0 0.129168 0.239761 0.239761 0.239761 0.239761
  spline S18 degree 3 poles (28.6358, -15.1755) (28.404, -14.9057) (27.9291, -14.3528) (27.8707, -13.6251) (27.8409, -13.2527) knots 0 0 0 0 0.103932 0.212913 0.212913 0.212913 0.212913
  spline S19 degree 3 poles (27.8409, -13.2527) (27.8706, -12.8914) (27.9288, -12.1834) (28.3925, -11.6465) (28.6197, -11.3836) knots 0 0 0 0 0.105739 0.207218 0.207218 0.207218 0.207218
  spline S20 degree 3 poles (28.6197, -11.3836) (28.9217, -11.1724) (29.5769, -10.7143) (30.3788, -10.678) (30.8111, -10.6585) knots 0 0 0 0 0.10836 0.235079 0.235079 0.235079 0.235079
  spline S21 degree 3 poles (30.8111, -10.6585) (30.8469, -10.6588) (30.9328, -10.6596) (31.0188, -10.6623) (31.0689, -10.6638) knots 0 0 0 0 0.010743 0.025787 0.025787 0.025787 0.025787
  line L29 (31.0689, -10.6638) -> (31.0689, -14.9177)
  spline S22 degree 3 poles (31.0689, -14.9177) (31.3553, -14.8898) (31.8837, -14.8383) (32.3121, -14.5281) (32.5083, -14.386) knots 0 0 0 0 0.084508 0.155921 0.155921 0.155921 0.155921
  spline S23 degree 3 poles (32.5083, -14.386) (32.654, -14.2157) (32.9481, -13.872) (32.9878, -13.4211) (33.0079, -13.1936) knots 0 0 0 0 0.065486 0.132192 0.132192 0.132192 0.132192
  spline S24 degree 3 poles (33.0079, -4.6321) (32.9979, -4.4636) (32.9786, -4.1379) (32.81, -3.859) (32.7286, -3.7244) knots 0 0 0 0 0.049772 0.096251 0.096251 0.096251 0.096251
  spline S25 degree 3 poles (32.7286, -3.7244) (32.6139, -3.603) (32.3629, -3.337) (32.0221, -3.2017) (31.837, -3.1282) knots 0 0 0 0 0.049501 0.108413 0.108413 0.108413 0.108413
  line L30 (31.837, -3.1282) -> (31.9605, -2.1292)
  spline S26 degree 3 poles (31.9605, -2.1292) (32.2331, -2.2209) (32.7605, -2.3986) (33.1373, -2.8072) (33.3194, -3.0046) knots 0 0 0 0 0.084738 0.163983 0.163983 0.163983 0.163983
  spline S27 degree 3 poles (33.3194, -3.0046) (33.4602, -3.2411) (33.7593, -3.7431) (33.7877, -4.328) (33.8028, -4.6375) knots 0 0 0 0 0.081309 0.172615 0.172615 0.172615 0.172615
  spline S28 degree 3 poles (33.8028, -4.6375) (33.7771, -5.0269) (33.7279, -5.7716) (33.2586, -6.3492) (33.0347, -6.6248) knots 0 0 0 0 0.113886 0.217791 0.217791 0.217791 0.217791
  spline S29 degree 3 poles (33.0347, -6.6248) (32.7361, -6.8375) (32.091, -7.2971) (31.2967, -7.3349) (30.8702, -7.3552) knots 0 0 0 0 0.107752 0.232763 0.232763 0.232763 0.232763
  spline S30 degree 3 poles (30.8702, -7.3552) (30.4295, -7.3351) (29.6116, -7.2978) (28.9438, -6.8299) (28.6358, -6.614) knots 0 0 0 0 0.129168 0.239761 0.239761 0.239761 0.239761
  spline S31 degree 3 poles (28.6358, -6.614) (28.404, -6.3441) (27.9291, -5.7912) (27.8707, -5.0636) (27.8409, -4.6912) knots 0 0 0 0 0.103932 0.212913 0.212913 0.212913 0.212913
  spline S32 degree 3 poles (27.8409, -4.6912) (27.8706, -4.3299) (27.9288, -3.6219) (28.3925, -3.085) (28.6197, -2.822) knots 0 0 0 0 0.105739 0.207218 0.207218 0.207218 0.207218
  spline S33 degree 3 poles (28.6197, -2.822) (28.9217, -2.6109) (29.5769, -2.1528) (30.3788, -2.1165) (30.8111, -2.0969) knots 0 0 0 0 0.10836 0.235079 0.235079 0.235079 0.235079
  spline S34 degree 3 poles (30.8111, -2.0969) (30.8469, -2.0973) (30.9328, -2.0981) (31.0188, -2.1008) (31.0689, -2.1023) knots 0 0 0 0 0.010743 0.025787 0.025787 0.025787 0.025787
  line L31 (31.0689, -2.1023) -> (31.0689, -6.3562)
  spline S35 degree 3 poles (31.0689, -6.3562) (31.3553, -6.3283) (31.8837, -6.2767) (32.3121, -5.9665) (32.5083, -5.8245) knots 0 0 0 0 0.084508 0.155921 0.155921 0.155921 0.155921
  spline S36 degree 3 poles (32.5083, -5.8245) (32.654, -5.6542) (32.9481, -5.3105) (32.9878, -4.8596) (33.0079, -4.6321) knots 0 0 0 0 0.065486 0.132192 0.132192 0.132192 0.132192
  spline S37 degree 3 poles (33.8028, 1.1365) (33.7932, 0.8013) (33.776, 0.1957) (33.4752, -0.3273) (33.3409, -0.5608) knots 0 0 0 0 0.098701 0.178335 0.178335 0.178335 0.178335
  spline S38 degree 3 poles (33.3409, -0.5608) (33.1602, -0.738) (32.7758, -1.115) (32.2499, -1.2372) (31.9712, -1.302) knots 0 0 0 0 0.074478 0.158426 0.158426 0.158426 0.158426
  line L32 (31.9712, -1.302) -> (31.8208, -0.346)
  spline S39 degree 3 poles (31.8208, -0.346) (31.9981, -0.3108) (32.3343, -0.2443) (32.5837, -0.0106) (32.7017, 0.0998) knots 0 0 0 0 0.052976 0.100497 0.100497 0.100497 0.100497
  spline S40 degree 3 poles (32.7017, 0.0998) (32.7908, 0.2436) (32.9858, 0.5582) (33.0001, 0.9295) (33.0079, 1.1311) knots 0 0 0 0 0.049907 0.109217 0.109217 0.109217 0.109217
  spline S41 degree 3 poles (33.0079, 1.1311) (33.0034, 1.3297) (32.9954, 1.6832) (32.8173, 1.9865) (32.7393, 2.1194) knots 0 0 0 0 0.058395 0.103914 0.103914 0.103914 0.103914
  spline S42 degree 3 poles (32.7393, 2.1194) (32.647, 2.2133) (32.4698, 2.3936) (32.2198, 2.4261) (32.1001, 2.4416) knots 0 0 0 0 0.038273 0.073449 0.073449 0.073449 0.073449
  spline S43 degree 3 poles (32.1001, 2.4416) (31.9964, 2.4292) (31.7863, 2.4041) (31.6523, 2.24) (31.5845, 2.157) knots 0 0 0 0 0.030125 0.060991 0.060991 0.060991 0.060991
  spline S44 degree 3 poles (31.5845, 2.157) (31.5331, 2.0424) (31.3904, 1.7247) (31.309, 1.3856) (31.2569, 1.1687) knots 0 0 0 0 0.037609 0.104304 0.104304 0.104304 0.104304
  spline S45 degree 3 poles (31.2569, 1.1687) (31.181, 0.866) (31.0553, 0.3645) (30.8689, -0.1174) (30.795, -0.3084) knots 0 0 0 0 0.093498 0.154885 0.154885 0.154885 0.154885
  spline S46 degree 3 poles (30.795, -0.3084) (30.7245, -0.4352) (30.5877, -0.6815) (30.3619, -0.8498) (30.2525, -0.9314) knots 0 0 0 0 0.042979 0.083454 0.083454 0.083454 0.083454
  spline S47 degree 3 poles (30.2525, -0.9314) (30.1327, -0.9925) (29.8912, -1.1156) (29.6207, -1.1324) (29.4844, -1.1409) knots 0 0 0 0 0.039882 0.080371 0.080371 0.080371 0.080371
  spline S48 degree 3 poles (29.4844, -1.1409) (29.3604, -1.134) (29.1151, -1.1205) (28.8914, -1.0191) (28.7808, -0.969) knots 0 0 0 0 0.036909 0.072993 0.072993 0.072993 0.072993
  spline S49 degree 3 poles (28.7808, -0.969) (28.6764, -0.9049) (28.4679, -0.7769) (28.3147, -0.5861) (28.2383, -0.491) knots 0 0 0 0 0.036467 0.072787 0.072787 0.072787 0.072787
  spline S50 degree 3 poles (28.2383, -0.491) (28.1837, -0.404) (28.0633, -0.2126) (27.9958, 0.0034) (27.959, 0.1213) knots 0 0 0 0 0.030679 0.06755 0.06755 0.06755 0.06755
  spline S51 degree 3 poles (27.959, 0.1213) (27.9246, 0.2558) (27.8541, 0.5307) (27.8453, 0.8143) (27.8409, 0.9592) knots 0 0 0 0 0.041509 0.084847 0.084847 0.084847 0.084847
  spline S52 degree 3 poles (27.8409, 0.9592) (27.847, 1.1708) (27.8586, 1.5719) (27.9779, 1.9547) (28.0342, 2.1355) knots 0 0 0 0 0.063161 0.119704 0.119704 0.119704 0.119704
  spline S53 degree 3 poles (28.0342, 2.1355) (28.0998, 2.2908) (28.2217, 2.5797) (28.4534, 2.7901) (28.5606, 2.8874) knots 0 0 0 0 0.049846 0.092769 0.092769 0.092769 0.092769
  spline S54 degree 3 poles (28.5606, 2.8874) (28.6858, 2.9627) (28.9587, 3.1269) (29.2719, 3.1876) (29.4414, 3.2205) knots 0 0 0 0 0.04349 0.094818 0.094818 0.094818 0.094818
  line L33 (29.4414, 3.2204) -> (29.5704, 2.2751)
  spline S55 degree 3 poles (29.5704, 2.2751) (29.433, 2.2451) (29.1666, 2.1868) (28.9754, 1.993) (28.8829, 1.8992) knots 0 0 0 0 0.041191 0.079875 0.079875 0.079875 0.079875
  spline S56 degree 3 poles (28.8829, 1.8992) (28.811, 1.7787) (28.6518, 1.5119) (28.6414, 1.2001) (28.6358, 1.029) knots 0 0 0 0 0.041435 0.091767 0.091767 0.091767 0.091767
  spline S57 degree 3 poles (28.6358, 1.029) (28.6373, 0.8345) (28.64, 0.4993) (28.7922, 0.2028) (28.856, 0.0784) knots 0 0 0 0 0.057333 0.098767 0.098767 0.098767 0.098767
  spline S58 degree 3 poles (28.856, 0.0784) (28.9294, -0.0046) (29.0682, -0.1614) (29.2744, -0.1919) (29.3716, -0.2063) knots 0 0 0 0 0.032048 0.06061 0.06061 0.06061 0.06061
  spline S59 degree 3 poles (29.3716, -0.2063) (29.4328, -0.2013) (29.5558, -0.1912) (29.6585, -0.1226) (29.71, -0.0881) knots 0 0 0 0 0.018102 0.036374 0.036374 0.036374 0.036374
  spline S60 degree 3 poles (29.71, -0.0881) (29.7609, -0.04) (29.8723, 0.0653) (29.9342, 0.206) (29.9678, 0.2825) knots 0 0 0 0 0.020804 0.045551 0.045551 0.045551 0.045551
  spline S61 degree 3 poles (29.9678, 0.2825) (29.9978, 0.3777) (30.0869, 0.6604) (30.1638, 0.9466) (30.2149, 1.1365) knots 0 0 0 0 0.029943 0.088911 0.088911 0.088911 0.088911
  spline S62 degree 3 poles (30.2149, 1.1365) (30.2924, 1.4284) (30.4207, 1.9117) (30.5964, 2.3798) (30.6661, 2.5652) knots 0 0 0 0 0.090525 0.149905 0.149905 0.149905 0.149905
  spline S63 degree 3 poles (30.6661, 2.5652) (30.7287, 2.6929) (30.8511, 2.9425) (31.066, 3.1184) (31.1709, 3.2043) knots 0 0 0 0 0.042122 0.082304 0.082304 0.082304 0.082304
  spline S64 degree 3 poles (31.1709, 3.2043) (31.2926, 3.2716) (31.5496, 3.4138) (31.8434, 3.4279) (31.9981, 3.4353) knots 0 0 0 0 0.041152 0.086904 0.086904 0.086904 0.086904
  spline S65 degree 3 poles (31.9981, 3.4353) (32.1582, 3.4226) (32.4839, 3.3969) (32.7671, 3.2336) (32.9112, 3.1506) knots 0 0 0 0 0.047533 0.09672 0.09672 0.09672 0.09672
  spline S66 degree 3 poles (32.9112, 3.1506) (33.0461, 3.044) (33.326, 2.8228) (33.4879, 2.5045) (33.5718, 2.3396) knots 0 0 0 0 0.050952 0.105714 0.105714 0.105714 0.105714
  spline S67 degree 3 poles (33.5718, 2.3396) (33.6392, 2.1526) (33.7791, 1.7639) (33.7947, 1.3508) (33.8028, 1.1365) knots 0 0 0 0 0.059253 0.123162 0.123162 0.123162 0.123162
  spline S68 degree 3 poles (33.545, 17.4914) (33.5825, 17.3004) (33.6647, 16.8821) (33.6706, 16.4556) (33.6739, 16.2239) knots 0 0 0 0 0.058278 0.12764 0.12764 0.12764 0.12764
  line L34 (33.6739, 16.2239) -> (33.6739, 13.2214)
  line L35 (33.6739, 13.2214) -> (25.7998, 13.2214)
  line L36 (25.7998, 13.2214) -> (25.7998, 16.1755)
  spline S69 degree 3 poles (25.7998, 16.1755) (25.8049, 16.449) (25.8139, 16.9434) (25.9713, 17.4113) (26.0415, 17.6204) knots 0 0 0 0 0.081462 0.147254 0.147254 0.147254 0.147254
  spline S70 degree 3 poles (26.0415, 17.6204) (26.1309, 17.7926) (26.3087, 18.1356) (26.6217, 18.3618) (26.7774, 18.4744) knots 0 0 0 0 0.057347 0.114135 0.114135 0.114135 0.114135
  spline S71 degree 3 poles (26.7774, 18.4744) (26.9423, 18.5652) (27.2657, 18.7434) (27.6336, 18.7719) (27.814, 18.7859) knots 0 0 0 0 0.055754 0.109362 0.109362 0.109362 0.109362
  spline S72 degree 3 poles (27.814, 18.7859) (27.9805, 18.774) (28.3167, 18.7501) (28.6144, 18.5918) (28.7647, 18.512) knots 0 0 0 0 0.049487 0.099919 0.099919 0.099919 0.099919
  spline S73 degree 3 poles (28.7647, 18.512) (28.9079, 18.4053) (29.2075, 18.1821) (29.3895, 17.8553) (29.4844, 17.6848) knots 0 0 0 0 0.052956 0.110758 0.110758 0.110758 0.110758
  spline S74 degree 3 poles (29.4844, 17.6848) (29.5626, 17.906) (29.7123, 18.3297) (30.0414, 18.6347) (30.1988, 18.7805) knots 0 0 0 0 0.069179 0.132554 0.132554 0.132554 0.132554
  spline S75 degree 3 poles (30.1988, 18.7805) (30.377, 18.8933) (30.7411, 19.1237) (31.1715, 19.1525) (31.3912, 19.1672) knots 0 0 0 0 0.062227 0.127135 0.127135 0.127135 0.127135
  spline S76 degree 3 poles (31.3912, 19.1672) (31.5716, 19.1578) (31.9292, 19.139) (32.2591, 18.9998) (32.4224, 18.9309) knots 0 0 0 0 0.053768 0.106518 0.106518 0.106518 0.106518
  spline S77 degree 3 poles (32.4224, 18.9309) (32.5684, 18.8525) (32.8459, 18.7036) (33.0542, 18.4679) (33.1529, 18.3562) knots 0 0 0 0 0.049262 0.093604 0.093604 0.093604 0.093604
  spline S78 degree 3 poles (33.1529, 18.3562) (33.2348, 18.2297) (33.4086, 17.9613) (33.4978, 17.654) (33.545, 17.4914) knots 0 0 0 0 0.044954 0.095403 0.095403 0.095403 0.095403
  spline S79 degree 3 poles (33.8028, 22.7927) (33.7751, 22.4168) (33.7216, 21.6887) (33.2587, 21.126) (33.0347, 20.8538) knots 0 0 0 0 0.11005 0.213174 0.213174 0.213174 0.213174
  spline S80 degree 3 poles (33.0347, 20.8538) (32.7329, 20.6395) (32.0735, 20.1715) (31.2619, 20.1367) (30.8218, 20.1179) knots 0 0 0 0 0.108767 0.23765 0.23765 0.23765 0.23765
  spline S81 degree 3 poles (30.8218, 20.1179) (30.3417, 20.1399) (29.4586, 20.1805) (28.783, 20.7424) (28.4746, 20.9988) knots 0 0 0 0 0.13965 0.256857 0.256857 0.256857 0.256857
  spline S82 degree 3 poles (28.4746, 20.9988) (28.2898, 21.2615) (27.9112, 21.7995) (27.8647, 22.4565) (27.8409, 22.7927) knots 0 0 0 0 0.094471 0.1935 0.1935 0.1935 0.1935
  spline S83 degree 3 poles (27.8409, 22.7927) (27.8697, 23.1636) (27.9259, 23.8869) (28.3888, 24.444) (28.6143, 24.7156) knots 0 0 0 0 0.108619 0.211858 0.211858 0.211858 0.211858
  spline S84 degree 3 poles (28.6143, 24.7156) (28.9083, 24.9331) (29.5378, 25.3989) (30.3228, 25.4401) (30.7412, 25.4621) knots 0 0 0 0 0.107339 0.229887 0.229887 0.229887 0.229887
  spline S85 degree 3 poles (30.7412, 25.4621) (31.0737, 25.4556) (31.6724, 25.4437) (32.2287, 25.226) (32.4761, 25.1291) knots 0 0 0 0 0.098777 0.177884 0.177884 0.177884 0.177884
  spline S86 degree 3 poles (32.4761, 25.1291) (32.6743, 25.0066) (33.0728, 24.7601) (33.3262, 24.3659) (33.4537, 24.1677) knots 0 0 0 0 0.068948 0.138665 0.138665 0.138665 0.138665
  spline S87 degree 3 poles (33.4537, 24.1677) (33.5555, 23.9521) (33.7612, 23.5166) (33.7888, 23.0356) (33.8028, 22.7927) knots 0 0 0 0 0.070815 0.143048 0.143048 0.143048 0.143048
  spline S88 degree 3 poles (33.8028, 6.6365) (33.7932, 6.3013) (33.776, 5.6957) (33.4752, 5.1727) (33.3409, 4.9392) knots 0 0 0 0 0.098701 0.178335 0.178335 0.178335 0.178335
  spline S89 degree 3 poles (33.3409, 4.9392) (33.1602, 4.762) (32.7758, 4.385) (32.2499, 4.2628) (31.9712, 4.198) knots 0 0 0 0 0.074478 0.158426 0.158426 0.158426 0.158426
  line L37 (31.9712, 4.198) -> (31.8208, 5.154)
  spline S90 degree 3 poles (31.8208, 5.154) (31.9981, 5.1891) (32.3343, 5.2557) (32.5837, 5.4894) (32.7017, 5.5998) knots 0 0 0 0 0.052976 0.100497 0.100497 0.100497 0.100497
  spline S91 degree 3 poles (32.7017, 5.5998) (32.7908, 5.7436) (32.9858, 6.0582) (33.0001, 6.4295) (33.0079, 6.6311) knots 0 0 0 0 0.049907 0.109217 0.109217 0.109217 0.109217
  spline S92 degree 3 poles (33.0079, 6.6311) (33.0034, 6.8297) (32.9954, 7.1832) (32.8173, 7.4865) (32.7393, 7.6194) knots 0 0 0 0 0.058395 0.103914 0.103914 0.103914 0.103914
  spline S93 degree 3 poles (32.7393, 7.6194) (32.647, 7.7133) (32.4698, 7.8936) (32.2198, 7.9261) (32.1001, 7.9416) knots 0 0 0 0 0.038273 0.073449 0.073449 0.073449 0.073449
  spline S94 degree 3 poles (32.1001, 7.9416) (31.9964, 7.9292) (31.7863, 7.9041) (31.6523, 7.74) (31.5845, 7.657) knots 0 0 0 0 0.030125 0.06099 0.06099 0.06099 0.06099
  spline S95 degree 3 poles (31.5845, 7.657) (31.5331, 7.5424) (31.3904, 7.2247) (31.309, 6.8856) (31.2569, 6.6687) knots 0 0 0 0 0.037609 0.104304 0.104304 0.104304 0.104304
  spline S96 degree 3 poles (31.2569, 6.6687) (31.181, 6.366) (31.0553, 5.8645) (30.8689, 5.3826) (30.795, 5.1916) knots 0 0 0 0 0.093498 0.154885 0.154885 0.154885 0.154885
  spline S97 degree 3 poles (30.795, 5.1916) (30.7245, 5.0648) (30.5877, 4.8185) (30.3619, 4.6502) (30.2525, 4.5686) knots 0 0 0 0 0.042979 0.083454 0.083454 0.083454 0.083454
  spline S98 degree 3 poles (30.2525, 4.5686) (30.1327, 4.5075) (29.8912, 4.3844) (29.6207, 4.3676) (29.4844, 4.3591) knots 0 0 0 0 0.039882 0.080371 0.080371 0.080371 0.080371
  spline S99 degree 3 poles (29.4844, 4.3591) (29.3604, 4.366) (29.1151, 4.3795) (28.8914, 4.4809) (28.7808, 4.531) knots 0 0 0 0 0.036909 0.072993 0.072993 0.072993 0.072993
  spline S100 degree 3 poles (28.7808, 4.531) (28.6764, 4.5951) (28.4679, 4.7231) (28.3147, 4.9139) (28.2383, 5.009) knots 0 0 0 0 0.036467 0.072787 0.072787 0.072787 0.072787
  spline S101 degree 3 poles (28.2383, 5.009) (28.1837, 5.096) (28.0633, 5.2874) (27.9958, 5.5034) (27.959, 5.6213) knots 0 0 0 0 0.030679 0.06755 0.06755 0.06755 0.06755
  spline S102 degree 3 poles (27.959, 5.6213) (27.9246, 5.7558) (27.8541, 6.0307) (27.8453, 6.3143) (27.8409, 6.4592) knots 0 0 0 0 0.041509 0.084847 0.084847 0.084847 0.084847
  spline S103 degree 3 poles (27.8409, 6.4592) (27.847, 6.6708) (27.8586, 7.0719) (27.9779, 7.4547) (28.0342, 7.6355) knots 0 0 0 0 0.063161 0.119704 0.119704 0.119704 0.119704
  spline S104 degree 3 poles (28.0342, 7.6355) (28.0998, 7.7908) (28.2217, 8.0797) (28.4534, 8.2901) (28.5606, 8.3874) knots 0 0 0 0 0.049846 0.092769 0.092769 0.092769 0.092769
  spline S105 degree 3 poles (28.5606, 8.3874) (28.6858, 8.4627) (28.9587, 8.6269) (29.2719, 8.6876) (29.4414, 8.7204) knots 0 0 0 0 0.04349 0.094818 0.094818 0.094818 0.094818
  line L38 (29.4414, 8.7204) -> (29.5704, 7.7751)
  spline S106 degree 3 poles (29.5704, 7.7751) (29.433, 7.7451) (29.1666, 7.6868) (28.9754, 7.493) (28.8829, 7.3992) knots 0 0 0 0 0.041191 0.079875 0.079875 0.079875 0.079875
  spline S107 degree 3 poles (28.8829, 7.3992) (28.811, 7.2787) (28.6518, 7.0119) (28.6414, 6.7001) (28.6358, 6.529) knots 0 0 0 0 0.041435 0.091767 0.091767 0.091767 0.091767
  spline S108 degree 3 poles (28.6358, 6.529) (28.6373, 6.3345) (28.64, 5.9993) (28.7922, 5.7028) (28.856, 5.5784) knots 0 0 0 0 0.057333 0.098767 0.098767 0.098767 0.098767